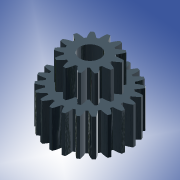
# Autodesk Inventor part: Spur Gear1
Saved by Autodesk Inventor 2017 (Build 210142000, 142)
## iProperties
Created: 2017-06-15
Part Number: Spur Gear1
Material: ABS Plastic
Document SubType Name: Modeling
Designer: zallen
Categories: <?xml version="1.0" encoding="UTF-16"?> <MemberInstance><Categories><FamilyTemplate><FamilyTemplateParameter ValueType="xs:double" Id="1" ObjectReferenceKey="da_z" ObjectType="kUserParameterObject"/><FamilyTemplateParameter ValueType="xs:double" Id="2" ObjectReferenceKey="da_b" ObjectType="kUserParameterObject"/><FamilyTemplateParameter ValueType="xs:double" Id="3" ObjectReferenceKey="da_beta" ObjectType="kUserParameterObject"/><FamilyTemplateParameter ValueType="xs:double" Id="4" ObjectReferenceKey="da_da" ObjectType="kUserParameterObject"/><FamilyTemplateParameter ValueType="xs:double" Id="5" ObjectReferenceKey="da_aw" ObjectType="kUserParameterObject"/><FamilyTemplateParameter ValueType="xs:string" Id="6" ObjectReferenceKey="EAIAABAAAACIAQAAAAAAAIAAAAAAAAAA" ObjectType="83910656" SubObjectId="SurfaceGeometry"/></FamilyTemplate><ParamToTemplateMap><ParamToTemplate CategoryParameter="//CategoryParameter[@InternalName='046C89C9-8512-4d59-83FE-43B91F4F132A']" TemplateParameter="1"/><ParamToTemplate CategoryParameter="//CategoryParameter[@InternalName='2552DF32-E462-4b46-AEBF-C6C7768E72AC']" TemplateParameter="2"/><ParamToTemplate CategoryParameter="//CategoryParameter[@InternalName='C9EE641D-15FC-4fae-A226-E94C4372FDD7']" TemplateParameter="3"/><ParamToTemplate><ParamToTemplate CategoryParameter="//CategoryParameter[@InternalName='00B6519A-459B-49c7-AD84-2E56D39A5744']" ConstantValue="0.000000"/></ParamToTemplate><ParamToTemplate><ParamToTemplate CategoryParameter="//CategoryParameter[@InternalName='04B31F0E-C7A6-4894-AA32-9629BEFACF47']" ConstantValue="1.000000"/></ParamToTemplate><ParamToTemplate><ParamToTemplate CategoryParameter="//CategoryParameter[@InternalName='43CBEC2E-7847-49e7-A936-2F7889FCB2D9']" ConstantValue="0.250000"/></ParamToTemplate><ParamToTemplate><ParamToTemplate CategoryParameter="//CategoryParameter[@InternalName='B1EFC894-105D-4ebd-86BF-FA20ED196853']" ConstantValue="0.350000"/></ParamToTemplate><ParamToTemplate><ParamToTemplate CategoryParameter="//CategoryParameter[@InternalName='51175063-3D10-4879-93E8-6246FE8B403D']" ConstantValue="2060000000.000000"/></ParamToTemplate><ParamToTemplate><ParamToTemplate CategoryParameter="//CategoryParameter[@InternalName='A3A52E27-4454-46a9-B0BD-C932399B70AF']" ConstantValue="0.300000"/></ParamToTemplate><ParamToTemplate><ParamToTemplate CategoryParameter="//CategoryParameter[@InternalName='91B76062-C214-41d9-B1B9-14D2AB99603D']" ConstantValue="0.177000"/></ParamToTemplate><ParamToTemplate><ParamToTemplate CategoryParameter="//CategoryParameter[@InternalName='374E806E-8B8A-4dda-A9AA-1039D6500AD2']" ConstantValue="5.649718"/></ParamToTemplate><ParamToTemplate><ParamToTemplate CategoryParameter="//CategoryParameter[@InternalName='2D373A89-B862-43d6-8D0B-0CBF12AB9F6C']" ConstantValue="0.349066"/></ParamToTemplate><ParamToTemplate CategoryParameter="//CategoryParameter[@InternalName='37777632-D6A2-4fac-9D53-DB8ACD95C989']" TemplateParameter="4"/><ParamToTemplate CategoryParameter="//CategoryParameter[@InternalName='FD1017F1-B727-4f7e-9707-0F86F1FF9423']" TemplateParameter="5"/><ParamToTemplate><ParamToTemplate CategoryParameter="//CategoryParameter[@InternalName='9E1B4470-B2D3-4ff1-B813-535BB4CDF51A']" ConstantValue="3520000.000000"/></ParamToTemplate><ParamToTemplate><ParamToTemplate CategoryParameter="//CategoryParameter[@InternalName='F8452263-BFF6-458c-9FB1-07C4B99E95CD']" ConstantValue="11400000.000000"/></ParamToTemplate><ParamToTemplate><ParamToTemplate CategoryParameter="//CategoryParameter[@InternalName='3E3BB259-FD49-497f-8171-6EBC954A3479']" ConstantValue="2.000000"/></ParamToTemplate><ParamToTemplate CategoryParameter="//CategoryParameter[@InternalName='27C3BAF2-7550-4e4b-AE2C-0DB134B7D9B7']" TemplateParameter="6"/></ParamToTemplateMap><Category DisplayName="Gear" InternalName="DC85795E-93AB-48d5-8EEE-5A27447B64BD" Mnemonic="Gear"><CategoryParameter DisplayName="z" InternalName="046C89C9-8512-4d59-83FE-43B91F4F132A" Mnemonic="z"/><CategoryParameter DisplayName="b" InternalName="2552DF32-E462-4b46-AEBF-C6C7768E72AC" Mnemonic="b"/><CategoryParameter DisplayName="||b|" InternalName="C9EE641D-15FC-4fae-A226-E94C4372FDD7" Mnemonic="beta"/><CategoryParameter DisplayName="x" InternalName="00B6519A-459B-49c7-AD84-2E56D39A5744" Mnemonic="x"/><CategoryParameter DisplayName="a*" InternalName="04B31F0E-C7A6-4894-AA32-9629BEFACF47" Mnemonic="a"/><CategoryParameter DisplayName="c*" InternalName="43CBEC2E-7847-49e7-A936-2F7889FCB2D9" Mnemonic="c"/><CategoryParameter DisplayName="r|.f|*" InternalName="B1EFC894-105D-4ebd-86BF-FA20ED196853" Mnemonic="rf"/><CategoryParameter DisplayName="E" InternalName="51175063-3D10-4879-93E8-6246FE8B403D" Mnemonic="E"/><CategoryParameter DisplayName="||m|" InternalName="A3A52E27-4454-46a9-B0BD-C932399B70AF" Mnemonic="mi"/><Category DisplayName="SpurGear" InternalName="26C5A22E-A91E-4dfd-A3B3-23CCAFAE1764" Mnemonic="SpurGear"><CategoryParameter DisplayName="m" InternalName="91B76062-C214-41d9-B1B9-14D2AB99603D" Mnemonic="m"/><CategoryParameter DisplayName="P" InternalName="374E806E-8B8A-4dda-A9AA-1039D6500AD2" Mnemonic="PP"/><CategoryParameter DisplayName="||a|" InternalName="2D373A89-B862-43d6-8D0B-0CBF12AB9F6C" Mnemonic="alpha"/><CategoryParameter DisplayName="d|.a|" InternalName="37777632-D6A2-4fac-9D53-DB8ACD95C989" Mnemonic="da"/><CategoryParameter DisplayName="a|.w|" InternalName="FD1017F1-B727-4f7e-9707-0F86F1FF9423" Mnemonic="aw"/><CategoryParameter DisplayName="||s||.Flim|" InternalName="9E1B4470-B2D3-4ff1-B813-535BB4CDF51A" Mnemonic="sFlim"/><CategoryParameter DisplayName="||s||.Hlim|" InternalName="F8452263-BFF6-458c-9FB1-07C4B99E95CD" Mnemonic="sHlim"/><CategoryParameter DisplayName="type" InternalName="3E3BB259-FD49-497f-8171-6EBC954A3479" Mnemonic="type"/><CategoryParameter DisplayName="PitchDiameter" InternalName="27C3BAF2-7550-4e4b-AE2C-0DB134B7D9B7" Mnemonic="IDS_PITCHDIAM"/></Category></Category></Categories></MemberInstance>
Density: 1.06 g/cm^3
Appearance: CR Dark Blue
CustomPartVersion: 1
Author: zallen
Autodesk Inventor part; units mm, degrees
sketch "Sketch1" plane through (0, 0, 0) normal (0, 0, 1) x (1, 0, 0)
  circle A0 centre (0, 0) radius 21.24
  dimension "d0" = 42.48
  constraints: 1 centre point
  measures "d0" diameter of A0
extrude "Extrusion1" add sketch "Sketch1" along normal blind 20
ref_plane "Work Plane2" through (0, 0, 10) normal (0, 0, 1) x (1, 0, 0)
sketch "Sketch2" plane through (0, 0, 0) normal (0, 0, -1) x (-1, 0, 0)
  circle A0 centre (0, 0) radius 21.24 projected
  circle A1 centre (0, 0) radius 19.4654
  dimension "d3" = 38.9309
  constraints: 1 centre point, 1 coincident
  measures "d3" diameter of A1
surface extrude "Pitch Diameter" sketch "Sketch2" against normal through all shown no curves A1
ref_plane "Work Plane8" through (0, 0, 0) normal (0.9898214, 0.1423148, 0) x (0, 0, 1)
ref_plane "Work Plane9" through (0, 0, 0) normal (1, 0, 0) x (0, 1, 0)
spur gear teeth "Spur Gear" teeth 22 pitch diameter 38.94 tip diameter 42.48 root diameter 34.515 face width 20 start plane through (0, 0, 0) normal (0, 0, -1) x (-1, 0, 0)
sketch "Sketch3" plane through (0, 0, 20) normal (0, 0, 1) x (1, 0, 0)
  circle A0 centre (0, 0) radius 5.5
  dimension "d49" = 11
  constraints: 1 centre point, 1 coincident
  measures "d49" diameter of A0
extrude "Extrusion2" cut sketch "Sketch3" against normal through all
sketch "Sketch4" plane through (0, 0, 0) normal (0, 0, -1) x (-1, 0, 0)
  arc A0 (0.7581, -21.2265) -> (1.8447, -17.1586) centre (-13.429, -15.2576) ccw projected
  arc A1 (-0.7581, -21.2265) -> (0.7581, -21.2265) centre (0, 0) ccw projected
  arc A2 (-1.8447, -17.1586) -> (-0.7581, -21.2265) centre (13.429, -15.2576) ccw projected
  arc A3 (1.8447, -17.1586) -> (3.0641, -16.9833) centre (0, 0) ccw projected
  arc A4 (0.7581, -21.2265) -> (1.8447, -17.1586) centre (-13.429, -15.2576) ccw
  arc A5 (-1.8447, -17.1586) -> (-0.7581, -21.2265) centre (13.429, -15.2576) ccw projected
  arc A6 (-1.8447, -17.1586) -> (-1.8447, -17.1586) centre (13.429, -15.2576) ccw
  arc A7 (-0.7581, -21.2265) -> (0.7581, -21.2265) centre (0, 0) ccw projected
  arc A8 (-0.7581, -21.2265) -> (0.7581, -21.2265) centre (0, 0) ccw
  arc A9 (0.7581, -13.8284) -> (1.8447, -9.8284) centre (-13.0351, -7.9337) ccw
  arc A10 (-0.7581, -13.8284) -> (0.7581, -13.8284) centre (0, 6.1573) ccw
  arc A11 (-1.8447, -9.8284) -> (-0.7581, -13.8284) centre (13.0351, -7.9337) ccw
  arc A12 (-1.8447, -9.8284) -> (1.8447, -9.8284) centre (0, 0) ccw
  circle A13 centre (0, 0) radius 5.5 projected
  arc A14 (2.934, -9.5599) -> (5.7551, -12.5967) centre (15.229, -0.9672) ccw
  arc A15 (2.934, -9.5599) -> (6.2009, -7.8453) centre (0, 0) ccw
  arc A16 (7.0976, -11.8921) -> (6.2009, -7.8453) centre (-7.855, -13.0827) ccw
  arc A17 (5.7551, -12.5967) -> (7.0976, -11.8921) centre (-2.8614, 5.452) ccw
  arc A18 (7.0407, -7.1013) -> (10.9499, -8.4793) centre (13.9341, 6.2208) ccw
  arc A19 (7.0407, -7.1013) -> (9.1365, -4.065) centre (0, 0) ccw
  arc A20 (11.8112, -7.2315) -> (9.1365, -4.065) centre (-0.8755, -15.2346) ccw
  arc A21 (10.9499, -8.4793) -> (11.8112, -7.2315) centre (-5.0673, 3.4977) ccw
  arc A22 (9.5344, -3.016) -> (13.6362, -2.4194) centre (9.4471, 11.9838) ccw
  arc A23 (9.5344, -3.016) -> (9.9791, 0.6466) centre (0, 0) ccw
  arc A24 (13.8189, -0.9142) -> (9.9791, 0.6466) centre (6.3047, -13.8964) ccw
  arc A25 (13.6362, -2.4194) -> (13.8189, -0.9142) centre (-6.1124, 0.7422) ccw
  arc A26 (9.8438, 1.7603) -> (13.1986, 4.1948) centre (2.7958, 15.0014) ccw
  arc A27 (9.8438, 1.7603) -> (8.5355, 5.2101) centre (0, 0) ccw
  arc A28 (12.6609, 5.6124) -> (8.5355, 5.2101) centre (12.0405, -9.3747) ccw
  arc A29 (13.1986, 4.1948) -> (12.6609, 5.6124) centre (-5.7571, -2.1834) ccw
  arc A30 (7.8982, 6.1334) -> (9.7374, 9.848) centre (-4.4959, 14.5824) ccw
  arc A31 (7.8982, 6.1334) -> (5.1366, 8.5799) centre (0, 0) ccw
  arc A32 (8.6025, 10.8534) -> (5.1366, 8.5799) centre (15.018, -2.7054) ccw
  arc A33 (9.7374, 9.848) -> (8.6025, 10.8534) centre (-4.083, -4.6088) ccw
  arc A34 (4.1432, 9.1013) -> (4.0454, 13.2451) centre (-10.7577, 10.8227) ccw
  arc A35 (4.1432, 9.1013) -> (0.5609, 9.9843) centre (0, 0) ccw
  arc A36 (2.5733, 13.608) -> (0.5609, 9.9843) centre (14.555, 4.5837) ccw
  arc A37 (4.0454, 13.2451) -> (2.5733, 13.608) centre (-1.4735, -5.9783) ccw
  arc A38 (-0.5609, 9.9843) -> (-2.5733, 13.608) centre (-14.555, 4.5837) ccw
  arc A39 (-0.5609, 9.9843) -> (-4.1432, 9.1013) centre (0, 0) ccw
  arc A40 (-4.0454, 13.2451) -> (-4.1432, 9.1013) centre (10.7577, 10.8227) ccw
  arc A41 (-2.5733, 13.608) -> (-4.0454, 13.2451) centre (1.4735, -5.9783) ccw
  arc A42 (-5.1366, 8.5799) -> (-8.6025, 10.8534) centre (-15.018, -2.7054) ccw
  arc A43 (-5.1366, 8.5799) -> (-7.8982, 6.1334) centre (0, 0) ccw
  arc A44 (-9.7374, 9.848) -> (-7.8982, 6.1334) centre (4.4959, 14.5824) ccw
  arc A45 (-8.6025, 10.8534) -> (-9.7374, 9.848) centre (4.083, -4.6088) ccw
  arc A46 (-8.5355, 5.2101) -> (-12.6609, 5.6124) centre (-12.0405, -9.3747) ccw
  arc A47 (-8.5355, 5.2101) -> (-9.8438, 1.7603) centre (0, 0) ccw
  arc A48 (-13.1986, 4.1948) -> (-9.8438, 1.7603) centre (-2.7958, 15.0014) ccw
  arc A49 (-12.6609, 5.6124) -> (-13.1986, 4.1948) centre (5.7571, -2.1834) ccw
  arc A50 (-9.9791, 0.6466) -> (-13.8189, -0.9142) centre (-6.3047, -13.8964) ccw
  arc A51 (-9.9791, 0.6466) -> (-9.5344, -3.016) centre (0, 0) ccw
  arc A52 (-13.6362, -2.4194) -> (-9.5344, -3.016) centre (-9.4471, 11.9838) ccw
  arc A53 (-13.8189, -0.9142) -> (-13.6362, -2.4194) centre (6.1124, 0.7422) ccw
  arc A54 (-9.1365, -4.065) -> (-11.8112, -7.2315) centre (0.8755, -15.2346) ccw
  arc A55 (-9.1365, -4.065) -> (-7.0407, -7.1013) centre (0, 0) ccw
  arc A56 (-10.9499, -8.4793) -> (-7.0407, -7.1013) centre (-13.9341, 6.2208) ccw
  arc A57 (-11.8112, -7.2315) -> (-10.9499, -8.4793) centre (5.0673, 3.4977) ccw
  arc A58 (-6.2009, -7.8453) -> (-7.0976, -11.8921) centre (7.855, -13.0827) ccw
  arc A59 (-6.2009, -7.8453) -> (-2.934, -9.5599) centre (0, 0) ccw
  arc A60 (-5.7551, -12.5967) -> (-2.934, -9.5599) centre (-15.229, -0.9672) ccw
  arc A61 (-7.0976, -11.8921) -> (-5.7551, -12.5967) centre (2.8614, 5.452) ccw
  circle A62 centre (0, 0) radius 10
  circle A63 centre (0, 0) radius 5.5
  point P0 (0, -13.8427)
  point P1 (6.433, -12.2571)
  point P2 (11.3924, -7.8636)
  point P3 (13.7418, -1.6686)
  point P4 (12.9432, 4.9087)
  point P5 (9.1794, 10.3614)
  point P6 (3.3128, 13.4405)
  point P7 (-3.3128, 13.4405)
  point P8 (-9.1794, 10.3614)
  point P9 (-12.9432, 4.9087)
  point P10 (-13.7418, -1.6686)
  point P11 (-11.3924, -7.8636)
  point P12 (-6.433, -12.2571)
  dimension "d53" = 15
  dimension "d54" = 20
  dimension "d55" = 4
  dimension "d58" = 15
  dimension "d59" = 4
  dimension "d60" = 10
  dimension "d63" = 360
  constraints: 109 point on circle, 56 centre point, 4 vertical alignment, 2 coincident, 2 concentric, 1 horizontal alignment, 175 other
  measures "d53" radius of A9
  measures "d54" radius of A10
  measures "d55" vertical distance of A9.start A9.end
  measures "d58" radius of A11
  measures "d59" vertical distance of A10.start A11.start
  measures "d60" radius of A12
extrude "Extrusion3" add sketch "Sketch4" against normal blind 35 contours A11 A12 A6 | A6 A12 A9 A10 A11 | A12 A62 A59 A55 A51 A47 A43 A39 A35 A31 A27 A23 A6 A13 | A6 A13 A23 A62 A19 A15 A12 | A24 A25 A22 A23 A6 | A6 A23 A24 | A60 A61 A58 A59 | A15 A16 A17 A14 | A27 A28 A29 A26 | A56 A57 A54 A55 | A20 A21 A18 A19 | A31 A32 A33 A30 | A52 A53 A50 A51 | A35 A36 A37 A34 | A48 A49 A46 A47 | A39 A40 A41 A38 | A44 A45 A42 A43
equation "\"d0\" = da_da"
equation "\"d1\" = da_b"
equation "\"d3\" = da_dw"
equation "\"d16\" = da_aw"
equation "\"d43\" = da_aw"
equation "\"d46\" = da_aw"
equation "\"da_da\" = 42.479976"
equation "\"da_b\" = 20"
equation "\"da_dw\" = 38.93086"
equation "\"da_aw\" = 58.396291"
body "Solid1"
body "Srf1"
